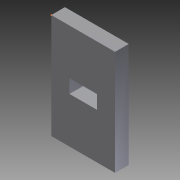
# Autodesk Inventor part: OpenROV 2_2 Horizontal Ducting Brace
Saved by Autodesk Inventor 2011 (Build 150239000, 239)
## iProperties
Created: 2011-12-03
Part Number: OpenROV 2_2 Horizontal Ducting Brace
Document SubType Name: Modeling
Designer: user
Density: 1 g/cm^3
Author: user
Autodesk Inventor part; units mm, degrees
ref_plane "YZ Plane" through (0, 0, 0) normal (1, 0, 0) x (0, 1, 0)
ref_plane "XZ Plane" through (0, 0, 0) normal (0, 1, 0) x (-1, 0, 0)
ref_plane "XY Plane" through (0, 0, 0) normal (0, 0, 1) x (1, 0, 0)
sketch "Sketch1" plane through (0, 0, 0) normal (0, 0, 1) x (1, 0, 0)
  point P0 (0, 0)
sketch "Sketch2" plane through (0, 0, 0) normal (0, 1, 0) x (-1, 0, 0)
  line L0 (0, 0) -> (-14, 0)
  line L1 (-14, 0) -> (-14, -23)
  line L2 (-14, -23) -> (0, -23)
  line L3 (0, -23) -> (0, 0)
  line L4 (-4, -13) -> (-10, -13)
  line L5 (-10, -13) -> (-10, -10)
  line L6 (-10, -10) -> (-4, -10)
  line L7 (-4, -10) -> (-4, -13)
  dimension "d0" = 14
  dimension "d1" = 23
  dimension "d2" = 6
  dimension "d3" = 3
  dimension "d4" = 10
  dimension "d5" = 4
  constraints: 16 end point, 4 parallel, 2 horizontal, 2 perpendicular
  measures "d0" distance of L0.start L0.end
  measures "d1" distance of L2.end L0.start
  measures "d2" distance of L4.start L4.end
  measures "d3" distance of L6.end L4.start
  measures "d4" distance between parallel lines of L0 L6
  measures "d5" distance between parallel lines of L3 L7
extrude "Extrusion1" add sketch "Sketch2" along normal blind 3
body "Solid1"
